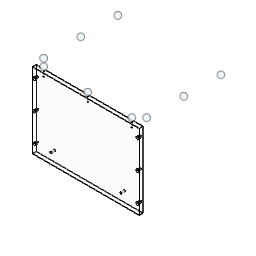
CAD_File 15 (Autodesk Fusion 360 design; units mm, degrees)
Autodesk Fusion 360 part; units mm, degrees
sketch "Sketch1" plane through (0, 0, 30) normal (0, 0, 1) x (-1, 0, 0)
  line L0 (-115, 107) -> (115, 107)
  line L1 (115, 107) -> (115, 115)
  line L2 (115, 115) -> (-115, 115)
  line L3 (-115, 115) -> (-115, 107)
  line L4 (115, 107) -> (-115, 107)
  line L5 (-115, 107) -> (-115, 115)
  line L6 (-115, 115) -> (115, 115)
  line L7 (115, 115) -> (115, 107)
  constraint horizontal L4
  constraint vertical L5
  constraint horizontal L6
  constraint vertical L7
  constraint coincident L2.end L3.start
  constraint coincident L0.end L1.start
extrude "Extrude1" add sketch "Sketch1" along normal up to surface (162 mm away)
sketch "Sketch2" plane through (0, -115, 0) normal (0, -1, 0) x (1, 0, 0)
  line L0 (115, 192) -> (-115, 192)
  line L1 (-115, 192) -> (-115, 30)
  line L2 (-115, 30) -> (115, 30)
  line L3 (115, 30) -> (115, 192)
  line L4 (0, 180) -> (0, 13.6981) construction
  circle A0 centre (-75.25, 52) radius 4
  circle A1 centre (75.25, 52) radius 4
  dimension "d834" = 8
  dimension "d835" = 8
  dimension "d836" = 75.25
  dimension "d837" = 140
  constraint perpendicular L2 L4
  constraint symmetric L4 A0 A1
  measures "d834" diameter of A0
  measures "d835" diameter of A1
  measures "d836" distance of L4 A0.centre
  measures "d837" distance of L0 A0.centre
extrude "Extrude2" cut sketch "Sketch2" against normal blind 8 contours A0 | A1
thread "Thread1" "ISO Metric profile 5.0 M5x0.8 6H" major diameter 5.12 minor diameter 4.234 pitch 0.8 angle 60 resizes the face on face at (-71.2699, -112.3333, 51.6017) on face at (79.2301, -112.3333, 51.6017)
sketch "Sketch3" plane through (0, -115, 0) normal (0, -1, 0) x (1, 0, 0)
  circle A0 centre (-75.25, 52) radius 2.117
  circle A1 centre (75.25, 52) radius 2.117
  line L0 (115, 192) -> (-115, 192)
  line L1 (-115, 192) -> (-115, 30)
  line L2 (-115, 30) -> (115, 30)
  line L3 (115, 30) -> (115, 192)
  line L4 (0, 210) -> (0, 20) construction
  line L5 (120, 111) -> (-120, 111) construction
  circle A2 centre (-111, 172) radius 1.5
  circle A3 centre (-111, 111) radius 1.5
  circle A4 centre (-111, 172) radius 3
  circle A5 centre (-111, 111) radius 3
  circle A6 centre (111, 172) radius 1.5
  circle A7 centre (111, 172) radius 3
  circle A8 centre (111, 111) radius 1.5
  circle A9 centre (111, 111) radius 3
  circle A10 centre (-111, 50) radius 1.5
  circle A11 centre (-111, 50) radius 3
  circle A12 centre (111, 50) radius 1.5
  circle A13 centre (111, 50) radius 3
  dimension "d896" = 81
  dimension "d897" = 3
  dimension "d898" = 4
  dimension "d899" = 20
  dimension "d901" = 3
  dimension "d902" = 4
  dimension "d903" = 6
  dimension "d904" = 6
  constraint perpendicular L2 L4
  constraint perpendicular L1 L5
  constraint coincident L5 A3.centre
  constraint concentric A2 A4
  constraint concentric A3 A5
  constraint symmetric L4 A2 A6
  constraint symmetric L4 A3 A8
  constraint symmetric L4 A4 A7
  constraint symmetric L4 A5 A9
  constraint symmetric L5 A2 A10
  constraint symmetric L5 A4 A11
  constraint symmetric L5 A6 A12
  constraint symmetric L5 A7 A13
  measures "d896" distance of L2 L5
  measures "d897" diameter of A2
  measures "d898" distance of L1 A2.centre
  measures "d899" distance of L0 A2.centre
  measures "d901" diameter of A3
  measures "d902" distance of L1 A3.centre
  measures "d903" diameter of A4
  measures "d904" diameter of A5
extrude "Extrude3" cut sketch "Sketch3" against normal blind 18 contours A2 | A3 | A6 | A8 | A10 | A12
extrude "Extrude4" cut sketch "Sketch3" against normal blind 3 contours A4 | A5 | A7 | A9 | A11 | A13
sketch "sketch 1014" plane through (0, 70, 200) normal (0, 0, 1) x (-1, 0, 0)
  circle A0 centre (111, 85) radius 1.5
  circle A1 centre (95, 181) radius 1.5
  circle A2 centre (-95, 181) radius 1.5
  circle A3 centre (-111, 85) radius 1.5
  circle A4 centre (-111, 5) radius 1.5
  circle A5 centre (-111, 165) radius 1.5
  circle A6 centre (0, 181) radius 1.5
  circle A7 centre (111, 165) radius 1.5
  circle A8 centre (111, 5) radius 1.5
extrude "Extrude5" cut sketch "sketch 1014" against normal blind 18
thread "Thread2" "ISO Metric profile 3.0 M3x0.5 6H" major diameter 3.086 minor diameter 2.529 pitch 0.5 angle 60 resizes the face on face at (-96.1957, -111.9057, 188.6667) on face at (96.1491, -111.9642, 185.3333) on face at (1.4095, -111.513, 185.3333)
